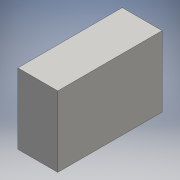
# Autodesk Inventor part: Receptor
Saved by Autodesk Inventor 2016 (Build 200138000, 138)
## iProperties
Created: 2019-03-15
Part Number: Receptor
Material: Genérico
Document SubType Name: Modeling
Designer: FIMCP
Density: 1 g/cm^3
Appearance: Valor por defecto
Mass: 10.166 g
Surface Area: 30.46 cm^2
Volume: 10.166 cm^3
Author: FIMCP
Autodesk Inventor part; units mm, degrees
ref_plane "YZ Plane" through (0, 0, 0) normal (1, 0, 0) x (0, 1, 0)
ref_plane "XZ Plane" through (0, 0, 0) normal (0, 1, 0) x (-1, 0, 0)
ref_plane "XY Plane" through (0, 0, 0) normal (0, 0, 1) x (1, 0, 0)
sketch "Boceto1" plane through (0, 0, 0) normal (1, 0, 0) x (0, 1, 0)
  line L0 (0, 0) -> (-34, 0)
  line L1 (-34, 0) -> (-34, -23)
  line L2 (-34, -23) -> (0, -23)
  line L3 (0, -23) -> (0, 0)
  dimension "d0" = 34
  dimension "d1" = 23
  constraints: 8 end point, 2 parallel, 1 horizontal, 1 perpendicular
  measures "d0" distance of L2.end L1.end
  measures "d1" distance of L1.end L0.end
extrude "Extrusión1" add sketch "Boceto1" along normal blind 13
